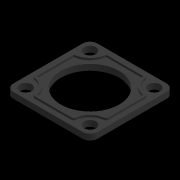
# Autodesk Inventor part: cnlink_5-pin_gasket_base
Saved by Autodesk Inventor 2020.2 (Build 242310000, 310)
## iProperties
Created: 2020-04-17
Part Number: cnlink_5-pin_gasket_base
Material: Rubber, Silicone
Document SubType Name: Modeling
Designer: agmlego
Mass: 0.252196 g
Surface Area: 5.19295 cm^2
Volume: 0.201757 cm^3
Density: 1.25 g/cm^3
Appearance: Rubber - Black
Author: agmlego
Autodesk Inventor part; units mm, degrees
ref_plane "YZ Plane" through (0, 0, 0) normal (1, 0, 0) x (0, 1, 0)
ref_plane "XZ Plane" through (0, 0, 0) normal (0, 1, 0) x (-1, 0, 0)
ref_plane "XY Plane" through (0, 0, 0) normal (0, 0, 1) x (1, 0, 0)
sketch "Sketch1" plane through (0, 0, 0) normal (0, 1, 0) x (-1, 0, 0)
  line L0 (0, 0) -> (17, 0)
  line L1 (17, 0) -> (17, -17)
  line L2 (17, -17) -> (0, -17)
  line L3 (0, -17) -> (0, 0)
  dimension "d0" = 17
  constraints: 8 end point, 2 parallel, 2 perpendicular, 1 horizontal
  measures "d0" distance of L0.start L0.end
extrude "Extrusion1" add sketch "Sketch1" along normal blind 1.2
fillet "Fillet1" radius 1.5 4 edges at (-17, 0.6, 0) (-17, 0.6, -17) (0, 0.6, -17) (0, 0.6, 0)
sketch "Sketch2" plane through (0, 1.2, 0) normal (0, 1, 0) x (1, 0, 0)
  circle A0 centre (-8.5, 8.5) radius 5.1932 construction
  line L0 (-15.5, 0) -> (-1.5, 0) construction
  line L1 (-8.5, 0) -> (-8.5, 17) construction
  line L2 (-1.5, 17) -> (-15.5, 17) construction
  line L3 (-15, 2) -> (-8.5, 8.5) construction
  arc A1 (-17, 1.5) -> (-15.5, 0) centre (-15.5, 1.5) ccw construction
  point P0 (0, 0)
  point P1 (-2, 2)
  point P2 (-2, 15)
  point P3 (-15, 15)
  dimension "d6" = 360
  dimension "d8" = 13
  constraints: 4 end point, 3 midpoint, 2 coincident, 1 centre point, 1 point on line, 5 other
  measures "d8" distance of point (-2, 2) L3.start
hole "Hole1" at (-15, 1.2, -15) at (-2, 1.2, -15) at (-2, 1.2, -2) at (-15, 1.2, -2) direction (0, -1, 0) diameter 2.4 end through all clearance for "Flat Head Machine Screw" size "M2" standard "Ansi Metric M Profile"
hole "Hole2" at (-8.5, 1.2, -8.5) direction (0, -1, 0) diameter 11.8 end through all
sketch "Sketch3" plane through (0, 1.2, 0) normal (0, 1, 0) x (1, 0, 0)
  line L0 (-12.1505, 1) -> (-4.8495, 1)
  line L1 (-1, 4.8495) -> (-1, 12.1505)
  line L2 (-4.8495, 16) -> (-12.1505, 16)
  line L3 (-16, 12.1505) -> (-16, 4.8495)
  line L4 (-16, 8.5) -> (-1, 8.5) construction
  line L5 (-8.5, 16) -> (-8.5, 1) construction
  circle A0 centre (-8.5, 8.5) radius 5.9 construction
  arc A1 (-12.7441, 1.5128) -> (-15.4872, 4.2559) centre (-15.9596, 1.0404) ccw
  arc A2 (-15.4872, 12.7441) -> (-12.7441, 15.4872) centre (-15.9596, 15.9596) ccw
  arc A3 (-4.2559, 15.4872) -> (-1.5128, 12.7441) centre (-1.0404, 15.9596) ccw
  arc A4 (-1.5128, 4.2559) -> (-4.2559, 1.5128) centre (-1.0404, 1.0404) ccw
  arc A5 (0, 15.5) -> (-1.5, 17) centre (-1.5, 15.5) ccw construction
  arc A6 (-12.7441, 1.5128) -> (-12.1505, 1) centre (-12.1505, 1.6) ccw
  arc A7 (-4.8495, 1) -> (-4.2559, 1.5128) centre (-4.8495, 1.6) ccw
  arc A8 (-1.5128, 4.2559) -> (-1, 4.8495) centre (-1.6, 4.8495) ccw
  arc A9 (-1, 12.1505) -> (-1.5128, 12.7441) centre (-1.6, 12.1505) ccw
  arc A10 (-4.2559, 15.4872) -> (-4.8495, 16) centre (-4.8495, 15.4) ccw
  arc A11 (-12.1505, 16) -> (-12.7441, 15.4872) centre (-12.1505, 15.4) ccw
  arc A12 (-15.4872, 12.7441) -> (-16, 12.1505) centre (-15.4, 12.1505) ccw
  arc A13 (-16, 4.8495) -> (-15.4872, 4.2559) centre (-15.4, 4.8495) ccw
  arc A14 (-4.8495, 1.5) -> (-4.7506, 1.5855) centre (-4.8495, 1.6) ccw
  arc A15 (-1.5855, 4.7506) -> (-4.7506, 1.5855) centre (-1.0404, 1.0404) ccw
  arc A16 (-1.5855, 4.7506) -> (-1.5, 4.8495) centre (-1.6, 4.8495) ccw
  line L6 (-1.5, 4.8495) -> (-1.5, 12.1505)
  arc A17 (-1.5, 12.1505) -> (-1.5855, 12.2494) centre (-1.6, 12.1505) ccw
  arc A18 (-4.7506, 15.4145) -> (-1.5855, 12.2494) centre (-1.0404, 15.9596) ccw
  arc A19 (-4.7506, 15.4145) -> (-4.8495, 15.5) centre (-4.8495, 15.4) ccw
  line L7 (-4.8495, 15.5) -> (-12.1505, 15.5)
  arc A20 (-12.1505, 15.5) -> (-12.2494, 15.4145) centre (-12.1505, 15.4) ccw
  arc A21 (-15.4145, 12.2494) -> (-12.2494, 15.4145) centre (-15.9596, 15.9596) ccw
  arc A22 (-15.4145, 12.2494) -> (-15.5, 12.1505) centre (-15.4, 12.1505) ccw
  line L8 (-15.5, 12.1505) -> (-15.5, 4.8495)
  arc A23 (-15.5, 4.8495) -> (-15.4145, 4.7506) centre (-15.4, 4.8495) ccw
  arc A24 (-12.2494, 1.5855) -> (-15.4145, 4.7506) centre (-15.9596, 1.0404) ccw
  arc A25 (-12.2494, 1.5855) -> (-12.1505, 1.5) centre (-12.1505, 1.6) ccw
  line L9 (-12.1505, 1.5) -> (-4.8495, 1.5)
  point P0 (0, 0)
  point P1 (-12.7099, 1)
  point P2 (-4.2901, 1)
  point P3 (-1, 4.2901)
  point P4 (-1, 12.7099)
  point P5 (-4.2901, 16)
  point P6 (-12.7099, 16)
  point P7 (-16, 12.7099)
  point P8 (-16, 4.2901)
  dimension "d23" = 15
  dimension "d24" = 3.25
  dimension "d26" = 4.1
  dimension "d27" = 0.6
  dimension "d28" = 0.5
  constraints: 56 point on circle, 24 centre point, 20 end point, 16 tangent, 10 equal radius, 8 point on line, 6 midpoint, 4 equal length, 3 coincident, 2 horizontal, 2 perpendicular, 2 vertical, 15 other
  measures "d23" distance between parallel lines of L1 L3
  measures "d24" radius of A1
  measures "d27" radius of A6
  measures "d28" distance between parallel lines of L0 L9
extrude "Extrusion2" add sketch "Sketch3" along normal blind 0.4
body "Solid1"
